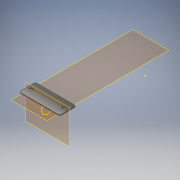
# Autodesk Inventor part: Plate
Saved by Autodesk Inventor 2019 (Build 230136000, 136)
## iProperties
Created: 2021-03-20
Part Number: Plate
Material: Steel, High Strength, Low Alloy
Document SubType Name: Modeling
Designer: rtavi
Density: 7.85 g/cm^3
Appearance: Steel - Polished
Author: rtavi
Autodesk Inventor part; units mm, degrees
ref_plane "YZ Plane" through (0, 0, 0) normal (1, 0, 0) x (0, 1, 0)
ref_plane "XY Plane" through (0, 0, 0) normal (0, 0, 1) x (1, 0, 0)
sketch "Sketch2" plane through (0, 0, 0) normal (1, 0, 0) x (0, 1, 0)
  circle A0 centre (27, 120) radius 7.5 projected
  line L0 (27, 120) -> (34.5, 120)
  point P0 (0, 0)
  constraints: 2 end point, 1 horizontal, 1 horizontal alignment, 1 other
ref_plane "Work Plane1" through (0, 34.5, 120) normal (0, 1, 0) x (-1, 0, 0)
sketch "Sketch3" plane through (0, 34.5, 120) normal (0, 1, 0) x (-1, 0, 0)
  line L0 (0, -120) -> (0, 59.5473) construction
  line L1 (-25, 10) -> (25, 10)
  line L2 (25, 10) -> (25, -10)
  line L3 (25, -10) -> (-25, -10)
  line L4 (-25, -10) -> (-25, 10)
  line L5 (-25, 0) -> (25, 0) construction
  point P0 (0, 0)
  point P1 (0, 0)
  point P2 (0, 0)
  dimension "d2" = 20
  dimension "d3" = 50
  constraints: 12 end point, 3 midpoint, 2 parallel, 1 horizontal, 1 perpendicular, 1 vertical, 1 other
  measures "d2" distance of L3.end L1.start
  measures "d3" distance of L1.start L1.end
extrude "Extrusion1" add sketch "Sketch3" along normal blind 1
sketch "Sketch4" plane through (0, 35.5, 120) normal (0, 1, 0) x (1, 0, 0)
  line L0 (25, -10) -> (25, 10) construction
  line L1 (25, 0) -> (-25, 0) construction
  line L2 (-25, 10) -> (-25, -10) construction
  line L3 (-25, -10) -> (25, -10) construction
  line L4 (20, -10) -> (20, 10) construction
  line L5 (25, 10) -> (-25, 10) construction
  line L6 (-20, -10) -> (-20, 10) construction
  point P0 (0, 120)
  point P1 (20, 0)
  point P2 (-20, 0)
  dimension "d6" = 5
  dimension "d7" = 5
  constraints: 6 end point, 4 midpoint, 4 point on line, 1 parallel, 1 perpendicular
  measures "d6" distance between parallel lines of L0 L4
  measures "d7" distance between parallel lines of L2 L6
hole "Hole1" at (20, 35.5, 120) at (-20, 35.5, 120) direction (0, -1, 0) diameter 4.1 end through all
fillet "Fillet1" radius 2 4 edges at (25, 35, 130) (25, 35, 110) (-25, 35, 130) (-25, 35, 110)
ref_plane "Work Plane2" through (-23, 34.5, 120) normal (0, 0, 1) x (1, 0, 0)
body "Solid1"
